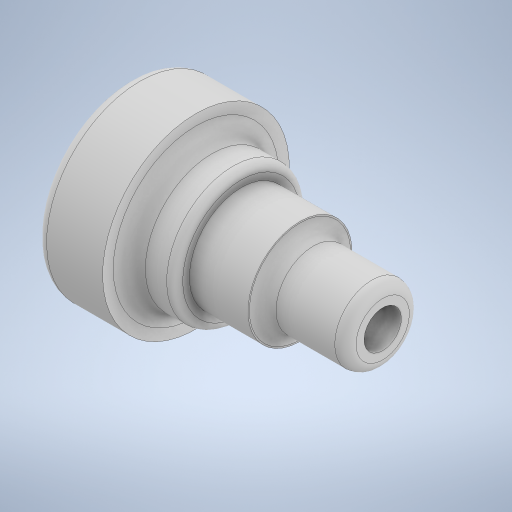
# Autodesk Inventor part: Bartosz_Zukowski_model_nr_9.ipj
Saved by Autodesk Inventor 2024 (Build 280153000, 153)
## iProperties
Created: 2024-04-11
Part Number: Bartosz_Zukowski_model_nr_9.ipj
Material: Ogólny
Document SubType Name: Modeling
Designer: Bartosz
Density: 1 g/cm^3
Appearance: Domyślna
Author: Bartosz
Autodesk Inventor part; units mm, degrees
ref_plane "YZ Plane" through (0, 0, 0) normal (1, 0, 0) x (0, 1, 0)
ref_plane "XZ Plane" through (0, 0, 0) normal (0, 1, 0) x (-1, 0, 0)
ref_plane "XY Plane" through (0, 0, 0) normal (0, 0, 1) x (1, 0, 0)
sketch "proba_1" plane through (0, 0, 0) normal (0, 0, 1) x (1, 0, 0)
  line L0 (0, 0) -> (0, 31)
  line L1 (4, 35) -> (25, 35)
  line L2 (25, 35) -> (25, 25)
  line L3 (25, 25) -> (39, 25)
  line L4 (42, 22) -> (42, 19.5)
  line L5 (42, 19.5) -> (64, 19.5)
  line L6 (64, 19.5) -> (64, 14)
  line L7 (64, 14) -> (91, 14)
  line L8 (95, 10) -> (95, 0)
  line L9 (95, 0) -> (0, 0)
  line L10 (0, 0) -> (0, -17)
  line L11 (0, -17) -> (17.0822, -17)
  line L12 (19.0822, -15) -> (19.0822, -13)
  line L13 (19.0822, -13) -> (39.8827, -13)
  line L14 (39.8827, -13) -> (39.8827, -7)
  line L15 (39.8827, -7) -> (95, -7)
  line L16 (95, -7) -> (95, 0)
  arc A0 (17.0822, -17) -> (19.0822, -15) centre (17.0822, -15) ccw
  arc A1 (4, 35) -> (0, 31) centre (4, 31) ccw
  arc A2 (95, 10) -> (91, 14) centre (91, 10) ccw
  arc A3 (42, 22) -> (39, 25) centre (39, 22) ccw
  dimension "d1" = 95
  dimension "d2" = 31
  dimension "d3" = 53
  dimension "d4" = 70
  dimension "d5" = 70
  dimension "d6" = 50
  dimension "d7" = 39
  dimension "d8" = 28
  dimension "d9" = 34
  dimension "d10" = 26
  dimension "d11" = 14
  dimension "d12" = 2
  dimension "d13" = 4
  dimension "d14" = 3
  constraints: 34 end point, 15 perpendicular, 8 point on circle, 8 tangent, 4 centre point, 2 vertical, 1 equal radius
  measures "d1" distance between parallel lines of L0 L8
  measures "d2" distance between parallel lines of L6 L8
  measures "d3" distance between parallel lines of L4 L8
  measures "d4" distance between parallel lines of L2 L8
  measures "d5" diameter of L1 L9
  measures "d6" diameter of L3 L9
  measures "d7" diameter of L5 L9
  measures "d8" diameter of L7 L9
  measures "d9" diameter of L11 L9
  measures "d10" diameter of L13 L9
  measures "d11" diameter of L15 L9
  measures "d12" radius of A0
  measures "d13" radius of A1
  measures "d14" radius of A3
revolve "Obrót1" add sketch "proba_1" angle 360 about axis through (95, 0, 0) along (-1, 0, 0) contours L0 A1 L1 L2 L3 A3 L4 L5 L6 L7 A2 L8 L9
revolve "Obrót2" cut sketch "proba_1" angle 360 about axis through (95, 0, 0) along (1, 0, 0) contours L9 L16 L15 L14 L13 L12 A0 L11 L10
fillet "Zaokrąglenie1" radius 6 1 edges at (25, -25, 0)
fillet "Zaokrąglenie2" radius 5 1 edges at (64, -14, 0)
chamfer "Faza1" distance 2 angle 45 1 edges at (0, 17, 0) measured on face at (0, 25.8684, 3.8291)
